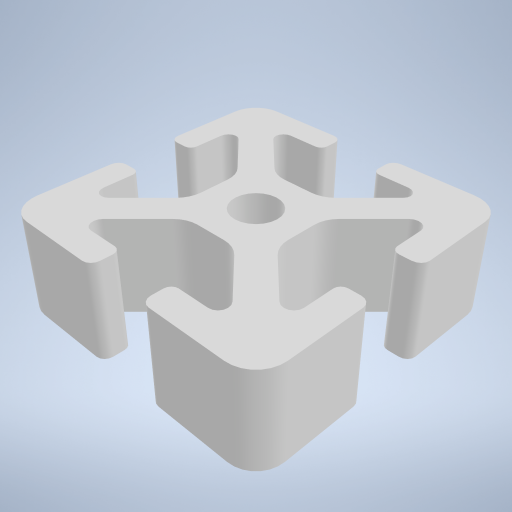
# Autodesk Inventor part: Item30x30
Saved by Autodesk Inventor 2024 (Build 280153020, 153B)
## iProperties
Created: 2023-08-17
Part Number: Item30x30
Material: Generisch
Document SubType Name: Modeling
Designer: hol
Density: 1 g/cm^3
Appearance: Vorgabe
Author: hol
Autodesk Inventor part; units mm, degrees
ref_plane "YZ Plane" through (0, 0, 0) normal (1, 0, 0) x (0, 1, 0)
ref_plane "XZ Plane" through (0, 0, 0) normal (0, 1, 0) x (-1, 0, 0)
ref_plane "XY Plane" through (0, 0, 0) normal (0, 0, 1) x (1, 0, 0)
sketch "Skizze1" plane through (0, 0, 0) normal (0, 0, 1) x (1, 0, 0)
  line L0 (25.2547, 7.1494) -> (21.1287, 11.2755)
  line L1 (8.8713, 18.7245) -> (4.7453, 22.8506)
  line L2 (22.8506, 4.7453) -> (18.7245, 8.8713)
  line L3 (11.2755, 21.1287) -> (7.1494, 25.2547)
  line L4 (19.1, 0) -> (27, 0)
  line L5 (3, 0) -> (10.9, 0)
  line L6 (7.8724, 3) -> (11.1, 3)
  line L7 (18.9, 3) -> (22.1276, 3)
  line L8 (13.3968, 9.75) -> (16.6032, 9.75)
  line L9 (27.8, 11.9) -> (29, 11.9)
  line L10 (1, 11.9) -> (2.2, 11.9)
  line L11 (27.8, 18.1) -> (29, 18.1)
  line L12 (1, 18.1) -> (2.2, 18.1)
  line L13 (13.3968, 20.25) -> (16.6032, 20.25)
  line L14 (18.9, 27) -> (22.1276, 27)
  line L15 (7.8724, 27) -> (11.1, 27)
  line L16 (19.1, 30) -> (27, 30)
  line L17 (3, 30) -> (10.9, 30)
  line L18 (21.1287, 18.7245) -> (25.2547, 22.8506)
  line L19 (7.1494, 4.7453) -> (11.2755, 8.8713)
  line L20 (18.7245, 21.1287) -> (22.8506, 25.2547)
  line L21 (4.7453, 7.1494) -> (8.8713, 11.2755)
  line L22 (0, 19.1) -> (0, 27)
  line L23 (0, 3) -> (0, 10.9)
  line L24 (3, 18.9) -> (3, 22.1276)
  line L25 (3, 7.8724) -> (3, 11.1)
  line L26 (9.75, 13.3968) -> (9.75, 16.6032)
  line L27 (11.9, 27.8) -> (11.9, 29)
  line L28 (11.9, 1) -> (11.9, 2.2)
  line L29 (18.1, 1) -> (18.1, 2.2)
  line L30 (18.1, 27.8) -> (18.1, 29)
  line L31 (20.25, 13.3968) -> (20.25, 16.6032)
  line L32 (27, 7.8724) -> (27, 11.1)
  line L33 (27, 18.9) -> (27, 22.1276)
  line L34 (30, 3) -> (30, 10.9)
  line L35 (30, 19.1) -> (30, 27)
  arc A0 (1, 11.9) -> (0, 10.9) centre (1, 10.9) ccw
  arc A1 (0, 19.1) -> (1, 18.1) centre (1, 19.1) ccw
  arc A2 (3, 11.1) -> (2.2, 11.9) centre (2.2, 11.1) ccw
  arc A3 (2.2, 18.1) -> (3, 18.9) centre (2.2, 18.9) ccw
  arc A4 (0, 3) -> (3, 0) centre (3, 3) ccw
  arc A5 (3, 30) -> (0, 27) centre (3, 27) ccw
  arc A6 (3, 7.8724) -> (4.7453, 7.1494) centre (4.0224, 7.8724) ccw
  arc A7 (4.7453, 22.8506) -> (3, 22.1276) centre (4.0224, 22.1276) ccw
  arc A8 (8.8713, 11.2755) -> (9.75, 13.3968) centre (6.75, 13.3968) ccw
  arc A9 (9.75, 16.6032) -> (8.8713, 18.7245) centre (6.75, 16.6032) ccw
  arc A10 (7.1494, 4.7453) -> (7.8724, 3) centre (7.8724, 4.0224) ccw
  arc A11 (7.8724, 27) -> (7.1494, 25.2547) centre (7.8724, 25.9776) ccw
  arc A12 (10.9, 0) -> (11.9, 1) centre (10.9, 1) ccw
  arc A13 (11.9, 29) -> (10.9, 30) centre (10.9, 29) ccw
  arc A14 (11.9, 2.2) -> (11.1, 3) centre (11.1, 2.2) ccw
  arc A15 (11.1, 27) -> (11.9, 27.8) centre (11.1, 27.8) ccw
  arc A16 (13.3968, 9.75) -> (11.2755, 8.8713) centre (13.3968, 6.75) ccw
  arc A17 (11.2755, 21.1287) -> (13.3968, 20.25) centre (13.3968, 23.25) ccw
  circle A18 centre (15, 15) radius 2.5
  arc A19 (18.7245, 8.8713) -> (16.6032, 9.75) centre (16.6032, 6.75) ccw
  arc A20 (16.6032, 20.25) -> (18.7245, 21.1287) centre (16.6032, 23.25) ccw
  arc A21 (18.9, 3) -> (18.1, 2.2) centre (18.9, 2.2) ccw
  arc A22 (18.1, 27.8) -> (18.9, 27) centre (18.9, 27.8) ccw
  arc A23 (18.1, 1) -> (19.1, 0) centre (19.1, 1) ccw
  arc A24 (19.1, 30) -> (18.1, 29) centre (19.1, 29) ccw
  arc A25 (22.1276, 3) -> (22.8506, 4.7453) centre (22.1276, 4.0224) ccw
  arc A26 (22.8506, 25.2547) -> (22.1276, 27) centre (22.1276, 25.9776) ccw
  arc A27 (20.25, 13.3968) -> (21.1287, 11.2755) centre (23.25, 13.3968) ccw
  arc A28 (21.1287, 18.7245) -> (20.25, 16.6032) centre (23.25, 16.6032) ccw
  arc A29 (25.2547, 7.1494) -> (27, 7.8724) centre (25.9776, 7.8724) ccw
  arc A30 (27, 22.1276) -> (25.2547, 22.8506) centre (25.9776, 22.1276) ccw
  arc A31 (27, 0) -> (30, 3) centre (27, 3) ccw
  arc A32 (30, 27) -> (27, 30) centre (27, 27) ccw
  arc A33 (27.8, 11.9) -> (27, 11.1) centre (27.8, 11.1) ccw
  arc A34 (27, 18.9) -> (27.8, 18.1) centre (27.8, 18.9) ccw
  arc A35 (30, 10.9) -> (29, 11.9) centre (29, 10.9) ccw
  arc A36 (29, 18.1) -> (30, 19.1) centre (29, 19.1) ccw
  point P0 (0, 0)
  point P1 (25.2547, 7.1494)
  point P2 (21.1287, 11.2755)
  point P3 (20.25, 16.6032)
  point P4 (21.1287, 18.7245)
  point P5 (25.2547, 22.8506)
  point P6 (27.8, 18.1)
  point P7 (18.1, 27.8)
  point P8 (22.8506, 25.2547)
  point P9 (18.7245, 21.1287)
  point P10 (16.6032, 20.25)
  point P11 (13.3968, 20.25)
  point P12 (11.2755, 21.1287)
  point P13 (7.1494, 25.2547)
  point P14 (8.8713, 18.7245)
  point P15 (8.8713, 11.2755)
  point P16 (4.7453, 7.1494)
  point P17 (7.8724, 3)
  point P18 (7.1494, 4.7453)
  point P19 (11.2755, 8.8713)
  point P20 (16.6032, 9.75)
  point P21 (18.7245, 8.8713)
  point P22 (22.8506, 4.7453)
  point P23 (27.8, 11.9)
  constraints: 72 end point, 72 point on circle, 37 centre point
extrude "Extrusion1" add sketch "Skizze1" along normal blind 10
